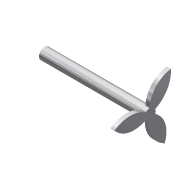
# Autodesk Inventor part: Motor Axle
Saved by Autodesk Inventor 2015 (Build 190159000, 159)
## iProperties
Created: 2015-04-16
Part Number: Motor Axle
Material: Generic
Document SubType Name: Modeling
Designer: jonathan
Density: 1 g/cm^3
Appearance: Default
Mass: 20.8242 g
Surface Area: 85.3325 cm^2
Volume: 20.8242 cm^3
Author: jonathan
Autodesk Inventor part; units mm, degrees
ref_plane "YZ Plane" through (0, 0, 0) normal (1, 0, 0) x (0, 1, 0)
ref_plane "XZ Plane" through (0, 0, 0) normal (0, 1, 0) x (-1, 0, 0)
ref_plane "XY Plane" through (0, 0, 0) normal (0, 0, 1) x (1, 0, 0)
sketch "Sketch1" plane through (0, 0, 0) normal (1, 0, 0) x (0, 1, 0)
  circle A0 centre (0, 0) radius 6.35
  dimension "d0" = 12.7
  constraints: 1 centre point, 1 coincident
  measures "d0" diameter of A0
extrude "Extrusion1" add sketch "Sketch1" along normal blind 127
sketch "Sketch2" plane through (127, 0, 0) normal (1, 0, 0) x (0, 0, -1)
  circle A0 centre (0, 0) radius 46.74
  constraints: 1 centre point, 1 coincident
extrude "Extrusion2" cut sketch "Sketch2" against normal blind 6.35
sketch "Sketch3" plane through (120.65, 0, 0) normal (1, 0, 0) x (0, 0, -1)
  arc A0 (0, 0) -> (23.8252, 33.0958) centre (-7.3529, 30.4168) ccw
  arc A1 (23.8252, 33.0958) -> (0, 0) centre (27.6846, 5.1939) ccw
  constraints: 4 point on circle, 2 centre point
extrude "Extrusion3" add sketch "Sketch3" against normal blind 4.7625
pattern_circular "Circular Pattern1" count 3 over 360 about axis through (0, 0, 0) along (1, 0, 0) of "Extrusion3"
body "Solid1"
